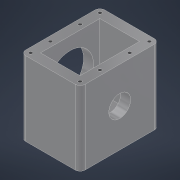
# Autodesk Inventor part: P016-Carter_corps
Saved by Autodesk Inventor 2021.3 (Build 253353000, 353)
## iProperties
Created: 2022-04-01
Part Number: P016-Carter_corps
Material: Aluminium
Document SubType Name: Modeling
Designer: remi
Density: 2.7 g/cm^3
Appearance: Aluminum - Dark
Mass: 820.09 g
Surface Area: 662.766 cm^2
Volume: 303.737 cm^3
Author: remi
Autodesk Inventor part; units mm, degrees
ref_plane "YZ Plane" through (0, 0, 0) normal (1, 0, 0) x (0, 1, 0)
ref_plane "XZ Plane" through (0, 0, 0) normal (0, 1, 0) x (-1, 0, 0)
ref_plane "XY Plane" through (0, 0, 0) normal (0, 0, 1) x (1, 0, 0)
sketch "Sketch2" plane through (0, 0, 0) normal (0, 0, 1) x (1, 0, 0)
  line L0 (-30, -40) -> (30, -40)
  line L1 (30, -40) -> (30, 40)
  line L2 (30, 40) -> (-30, 40)
  line L3 (-30, 40) -> (-30, -40)
  line L4 (-30, -40) -> (30, 40) construction
  line L5 (30, -40) -> (-30, 40) construction
  line L6 (20, -30) -> (-20, -30)
  line L7 (-20, -30) -> (-20, 30)
  line L8 (-20, 30) -> (20, 30)
  line L9 (20, 30) -> (20, -30)
  line L10 (20, -30) -> (-20, 30) construction
  line L11 (-20, -30) -> (20, 30) construction
  point P0 (0, 0)
  dimension "d0" = 60
  dimension "d1" = 10
  dimension "d2" = 10
  dimension "d3" = 60
  constraints: 24 end point, 4 midpoint, 4 parallel, 2 horizontal, 2 perpendicular
  measures "d0" distance of L1.end L2.end
  measures "d1" distance between parallel lines of L3 L7
  measures "d2" distance between parallel lines of L2 L8
  measures "d3" distance of L6.end L7.end
extrude "Extrusion1" add sketch "Sketch2" along normal blind 65
sketch "Sketch3" plane through (0, 0, 0) normal (0, 0, -1) x (-1, 0, 0)
  line L0 (-30, -40) -> (-30, 40) projected
  line L1 (30, -40) -> (-30, -40) projected
  line L2 (30, 40) -> (30, -40) projected
  line L3 (-30, 40) -> (30, 40) projected
  line L4 (-20, -30) -> (20, -30) construction
  line L5 (-20, 30) -> (-20, -30) construction
  line L6 (20, 30) -> (-20, 30) construction
  line L7 (20, -30) -> (20, 30) construction
  point P0 (0, 0)
extrude "Extrusion2" add sketch "Sketch3" along normal blind 10
sketch "Sketch4" plane through (30, -40, 65) normal (1, 0, 0) x (0, 0, -1)
  line L0 (75, 80) -> (0, 80) construction
  line L1 (0, 0) -> (0, 80) construction
  line L2 (0, 0) -> (75, 0) construction
  line L3 (75, 80) -> (75, 0) construction
  line L4 (75, 80) -> (75, 0) construction
  line L5 (65, 70) -> (65, 10) construction
  line L6 (65, 10) -> (0, 10) construction
  line L7 (0, 70) -> (0, 10) construction
  line L8 (65, 70) -> (0, 70) construction
  line L9 (0, 10) -> (65, 70) construction
  line L10 (0, 70) -> (65, 10) construction
  point P0 (65, 40)
  point P1 (36.5, 40)
  point P2 (32.5, 40)
  point P3 (32.5, 40)
  dimension "d22" = 4
  constraints: 4 end point, 2 midpoint, 1 horizontal alignment
  measures "d22" distance of point (32.5, 40) point (36.5, 40)
hole "Hole1" at (30, 0, 28.5) direction (-1, 0, 0) diameter 22 depth 10
sketch "Sketch5" plane through (0, 0, 65) normal (0, 0, 1) x (1, 0, 0)
  line L0 (30, -40) -> (30, 40) construction
  line L1 (30, 40) -> (-30, 40) construction
  line L2 (-30, 40) -> (-30, -40) construction
  line L3 (-30, -40) -> (30, -40) construction
  line L4 (20, -30) -> (-20, -30) construction
  line L5 (-20, -30) -> (-20, 30) construction
  line L6 (-20, 30) -> (20, 30) construction
  line L7 (20, 30) -> (20, -30) construction
  line L8 (-25, -35) -> (25, -35) construction
  line L9 (25, 35) -> (-25, 35) construction
  line L10 (-25, -35) -> (25, 35) construction
  line L11 (25, -35) -> (-25, 35) construction
  line L12 (-20, 30) -> (-25, 35) construction
  line L13 (-25, 35) -> (-30, 40) construction
  line L14 (-25, 35) -> (-25, 15) construction
  line L15 (-25, -15) -> (-25, -35) construction
  line L16 (25, -35) -> (25, -15) construction
  line L17 (25, 15) -> (25, 35) construction
  line L18 (-30, 40) -> (-30, -40) construction
  line L19 (-20, -30) -> (-20, 30) construction
  point P0 (0, 0)
  dimension "d24" = 20
  dimension "d26" = 30
  constraints: 20 end point, 8 coincident, 6 collinear, 3 parallel, 2 midpoint, 1 horizontal, 1 horizontal alignment, 1 perpendicular
  measures "d24" distance of L15.start L15.end
  measures "d26" distance of point (-25, 15) point (-25, -15)
hole "Hole2" at (25, -35, 65) at (-25, -35, 65) at (-25, 35, 65) at (25, 35, 65) at (-25, 15, 65) at (-25, -15, 65) at (25, -15, 65) at (25, 15, 65) direction (0, 0, -1) diameter 3.242 depth 10 thread size "M4x0.7" class "6H" standard "ISO Metric profile"
fillet "Fillet1" radius 5 4 edges at (30, -40, 27.5) (30, 40, 27.5) (-30, 40, 27.5) (-30, -40, 27.5)
sketch "Sketch6" plane through (-30, -35, 65) normal (-1, 0, 0) x (0, 0, 1)
  circle A0 centre (-36.5, 35) radius 11 construction
  circle A1 centre (-36.5, 35) radius 11 construction
  circle A2 centre (-36.5, 35) radius 23.5
  line L0 (-65, 5) -> (-65, 65) construction
  line L1 (-60, 56.0669) -> (-60, 13.1664) construction
  point P0 (-65, 35)
  dimension "d27" = 5
  dimension "d30" = 47
  constraints: 2 end point, 1 centre point, 1 coincident, 1 tangent, 1 vertical
  measures "d27" distance between parallel lines of L0 L1
  measures "d30" diameter of A2
extrude "Extrusion3" cut sketch "Sketch6" against normal up to surface (10 mm away)
sketch "Sketch9" plane through (-30, -35, 65) normal (-1, 0, 0) x (0, 0, 1)
  circle A0 centre (-36.5, 35) radius 30 construction
  circle A1 centre (-36.5, 35) radius 23.5 construction
  circle A2 centre (-36.5, 35) radius 11 construction
  circle A3 centre (-36.5, 35) radius 26.75 construction
  circle A4 centre (-49.875, 58.1662) radius 2.25 projected
  circle A5 centre (-49.875, 11.8338) radius 2.25 projected
  circle A6 centre (-9.75, 35) radius 2.25 projected
  circle A7 centre (-23.125, 11.8338) radius 2.25 projected
  circle A8 centre (-63.25, 35) radius 2.25 projected
  circle A9 centre (-23.125, 58.1662) radius 2.25 projected
  point P0 (-65, 35)
  point P1 (-9.75, 35)
  point P2 (-23.125, 58.1662)
  point P3 (-49.875, 58.1662)
  point P4 (-63.25, 35)
  point P5 (-49.875, 11.8338)
  point P6 (-23.125, 11.8338)
  dimension "d39" = 60
  dimension "d40" = 53.5
  dimension "d38" = 47
  dimension "d43" = 360
  constraints: 3 horizontal alignment, 1 coincident, 9 other
  measures "d38" diameter of A1
hole "Hole4" at (-30, -23.1662, 41.875) at (-30, -23.1662, 15.125) at (-30, 0, 1.75) at (-30, 23.1662, 15.125) at (-30, 23.1662, 41.875) at (-30, 0, 55.25) direction (1, 0, 0) diameter 3.242 depth 6 tip angle 118 start extended yes thread size "M4x0.7" class "6H" standard "ISO Metric profile"
equation "\"d2\" = d1"
equation "\"d3\" = d0"
equation "\"d26\" = 1.5 * d24"
equation "\"d40\" = 0.5 * d39 + 0.5 * d38"
body "Solid1"
